Autodesk Fusion 360 part; units mm, degrees
(part 3 of 5)
  line L1736 (93.1413, -105.9405) -> (93.1413, -102.4186)
  line L1737 (93.1413, -102.4186) -> (79.4991, -102.4186)
  line L1738 (112.2258, -102.3705) -> (112.2394, -102.3841)
  line L1739 (112.2394, -102.3841) -> (112.2413, -102.3936)
  line L1740 (112.2413, -102.3936) -> (112.2413, -105.9655)
  line L1741 (112.2413, -105.9655) -> (112.2394, -105.9751)
  line L1742 (112.2394, -105.9751) -> (112.2258, -105.9886)
  line L1743 (112.2258, -105.9886) -> (112.2163, -105.9905)
  line L1744 (112.2163, -105.9905) -> (109.86, -105.9905)
  line L1745 (109.86, -105.9905) -> (109.86, -106.8585)
  line L1746 (109.86, -106.8585) -> (109.8581, -106.868)
  line L1747 (109.8581, -106.868) -> (109.8446, -106.8816)
  line L1748 (109.8446, -106.8816) -> (109.835, -106.8835)
  line L1749 (109.835, -106.8835) -> (107.1811, -106.8835)
  line L1750 (107.1811, -106.8835) -> (107.1811, -110.728)
  line L1751 (107.1811, -110.728) -> (107.1811, -111.9186)
  line L1752 (107.1811, -111.9186) -> (107.1792, -111.9282)
  line L1753 (107.1792, -111.9282) -> (107.1657, -111.9417)
  line L1754 (107.1657, -111.9417) -> (107.1561, -111.9436)
  line L1755 (107.1561, -111.9436) -> (102.6913, -111.9436)
  line L1756 (102.6913, -111.9436) -> (102.3936, -111.9436)
  line L1757 (102.3936, -111.9436) -> (102.384, -111.9417)
  line L1758 (102.384, -111.9417) -> (102.3705, -111.9282)
  line L1759 (102.3705, -111.9282) -> (102.3686, -111.9186)
  line L1760 (102.3686, -111.9186) -> (102.3686, -108.9671)
  line L1761 (102.3686, -108.9671) -> (100.9303, -108.9671)
  line L1762 (100.9303, -108.9671) -> (100.9303, -110.728)
  line L1763 (100.9303, -110.728) -> (100.9284, -110.7376)
  line L1764 (100.9284, -110.7376) -> (100.9149, -110.7511)
  line L1765 (100.9149, -110.7511) -> (100.9053, -110.753)
  line L1766 (100.9053, -110.753) -> (98.5241, -110.753)
  line L1767 (98.5241, -110.753) -> (98.5145, -110.7511)
  line L1768 (98.5145, -110.7511) -> (98.501, -110.7376)
  line L1769 (98.501, -110.7376) -> (98.4991, -110.728)
  line L1770 (98.4991, -110.728) -> (98.4991, -108.6694)
  line L1771 (98.4991, -108.6694) -> (96.1428, -108.6694)
  line L1772 (96.1428, -108.6694) -> (96.1333, -108.6675)
  line L1773 (96.1333, -108.6675) -> (96.1197, -108.654)
  line L1774 (96.1197, -108.654) -> (96.1178, -108.6444)
  line L1775 (96.1178, -108.6444) -> (96.1178, -105.3702)
  line L1776 (96.1178, -105.3702) -> (96.1197, -105.3606)
  line L1777 (96.1197, -105.3606) -> (96.1333, -105.3471)
  line L1778 (96.1333, -105.3471) -> (96.1428, -105.3452)
  line L1779 (96.1428, -105.3452) -> (98.4991, -105.3452)
  line L1780 (98.4991, -105.3452) -> (98.4991, -102.3936)
  line L1781 (98.4991, -102.3936) -> (98.501, -102.3841)
  line L1782 (98.501, -102.3841) -> (98.5145, -102.3705)
  line L1783 (98.5145, -102.3705) -> (98.5241, -102.3686)
  line L1784 (98.5241, -102.3686) -> (112.2163, -102.3686)
  line L1785 (112.2163, -102.3686) -> (112.2258, -102.3705)
  line L1786 (98.5491, -102.4186) -> (98.5491, -105.3702)
  line L1787 (98.5491, -105.3702) -> (98.5472, -105.3798)
  line L1788 (98.5472, -105.3798) -> (98.5336, -105.3933)
  line L1789 (98.5336, -105.3933) -> (98.5241, -105.3952)
  line L1790 (98.5241, -105.3952) -> (96.1678, -105.3952)
  line L1791 (96.1678, -105.3952) -> (96.1678, -108.6194)
  line L1792 (96.1678, -108.6194) -> (98.5241, -108.6194)
  line L1793 (98.5241, -108.6194) -> (98.5336, -108.6213)
  line L1794 (98.5336, -108.6213) -> (98.5472, -108.6348)
  line L1795 (98.5472, -108.6348) -> (98.5491, -108.6444)
  line L1796 (98.5491, -108.6444) -> (98.5491, -110.703)
  line L1797 (98.5491, -110.703) -> (100.8803, -110.703)
  line L1798 (100.8803, -110.703) -> (100.8803, -108.9421)
  line L1799 (100.8803, -108.9421) -> (100.8822, -108.9325)
  line L1800 (100.8822, -108.9325) -> (100.8958, -108.919)
  line L1801 (100.8958, -108.919) -> (100.9053, -108.9171)
  line L1802 (100.9053, -108.9171) -> (102.3936, -108.9171)
  line L1803 (102.3936, -108.9171) -> (102.4032, -108.919)
  line L1804 (102.4032, -108.919) -> (102.4167, -108.9325)
  line L1805 (102.4167, -108.9325) -> (102.4186, -108.9421)
  line L1806 (102.4186, -108.9421) -> (102.4186, -111.8936)
  line L1807 (102.4186, -111.8936) -> (102.6913, -111.8936)
  line L1808 (102.6913, -111.8936) -> (107.1311, -111.8936)
  line L1809 (107.1311, -111.8936) -> (107.1311, -110.728)
  line L1810 (107.1311, -110.728) -> (107.1311, -106.8585)
  line L1811 (107.1311, -106.8585) -> (107.133, -106.8489)
  line L1812 (107.133, -106.8489) -> (107.1465, -106.8354)
  line L1813 (107.1465, -106.8354) -> (107.1561, -106.8335)
  line L1814 (107.1561, -106.8335) -> (109.81, -106.8335)
  line L1815 (109.81, -106.8335) -> (109.81, -105.9655)
  line L1816 (109.81, -105.9655) -> (109.8119, -105.9559)
  line L1817 (109.8119, -105.9559) -> (109.8254, -105.9424)
  line L1818 (109.8254, -105.9424) -> (109.835, -105.9405)
  line L1819 (109.835, -105.9405) -> (112.1913, -105.9405)
  line L1820 (112.1913, -105.9405) -> (112.1913, -102.4186)
  line L1821 (112.1913, -102.4186) -> (98.5491, -102.4186)
  line L1822 (131.2758, -102.3705) -> (131.2894, -102.3841)
  line L1823 (131.2894, -102.3841) -> (131.2913, -102.3936)
  line L1824 (131.2913, -102.3936) -> (131.2913, -105.9655)
  line L1825 (131.2913, -105.9655) -> (131.2894, -105.9751)
  line L1826 (131.2894, -105.9751) -> (131.2758, -105.9886)
  line L1827 (131.2758, -105.9886) -> (131.2663, -105.9905)
  line L1828 (131.2663, -105.9905) -> (128.91, -105.9905)
  line L1829 (128.91, -105.9905) -> (128.91, -106.8585)
  line L1830 (128.91, -106.8585) -> (128.9081, -106.868)
  line L1831 (128.9081, -106.868) -> (128.8946, -106.8816)
  line L1832 (128.8946, -106.8816) -> (128.885, -106.8835)
  line L1833 (128.885, -106.8835) -> (126.2311, -106.8835)
  line L1834 (126.2311, -106.8835) -> (126.2311, -110.728)
  line L1835 (126.2311, -110.728) -> (126.2311, -111.9186)
  line L1836 (126.2311, -111.9186) -> (126.2292, -111.9282)
  line L1837 (126.2292, -111.9282) -> (126.2157, -111.9417)
  line L1838 (126.2157, -111.9417) -> (126.2061, -111.9436)
  line L1839 (126.2061, -111.9436) -> (121.7413, -111.9436)
  line L1840 (121.7413, -111.9436) -> (121.4436, -111.9436)
  line L1841 (121.4436, -111.9436) -> (121.434, -111.9417)
  line L1842 (121.434, -111.9417) -> (121.4205, -111.9282)
  line L1843 (121.4205, -111.9282) -> (121.4186, -111.9186)
  line L1844 (121.4186, -111.9186) -> (121.4186, -108.9671)
  line L1845 (121.4186, -108.9671) -> (119.9803, -108.9671)
  line L1846 (119.9803, -108.9671) -> (119.9803, -110.728)
  line L1847 (119.9803, -110.728) -> (119.9784, -110.7376)
  line L1848 (119.9784, -110.7376) -> (119.9649, -110.7511)
  line L1849 (119.9649, -110.7511) -> (119.9553, -110.753)
  line L1850 (119.9553, -110.753) -> (117.5741, -110.753)
  line L1851 (117.5741, -110.753) -> (117.5645, -110.7511)
  line L1852 (117.5645, -110.7511) -> (117.551, -110.7376)
  line L1853 (117.551, -110.7376) -> (117.5491, -110.728)
  line L1854 (117.5491, -110.728) -> (117.5491, -108.6694)
  line L1855 (117.5491, -108.6694) -> (115.1928, -108.6694)
  line L1856 (115.1928, -108.6694) -> (115.1833, -108.6675)
  line L1857 (115.1833, -108.6675) -> (115.1697, -108.654)
  line L1858 (115.1697, -108.654) -> (115.1678, -108.6444)
  line L1859 (115.1678, -108.6444) -> (115.1678, -105.3702)
  line L1860 (115.1678, -105.3702) -> (115.1697, -105.3606)
  line L1861 (115.1697, -105.3606) -> (115.1833, -105.3471)
  line L1862 (115.1833, -105.3471) -> (115.1928, -105.3452)
  line L1863 (115.1928, -105.3452) -> (117.5491, -105.3452)
  line L1864 (117.5491, -105.3452) -> (117.5491, -102.3936)
  line L1865 (117.5491, -102.3936) -> (117.551, -102.3841)
  line L1866 (117.551, -102.3841) -> (117.5645, -102.3705)
  line L1867 (117.5645, -102.3705) -> (117.5741, -102.3686)
  line L1868 (117.5741, -102.3686) -> (131.2663, -102.3686)
  line L1869 (131.2663, -102.3686) -> (131.2758, -102.3705)
  line L1870 (117.5991, -102.4186) -> (117.5991, -105.3702)
  line L1871 (117.5991, -105.3702) -> (117.5972, -105.3798)
  line L1872 (117.5972, -105.3798) -> (117.5836, -105.3933)
  line L1873 (117.5836, -105.3933) -> (117.5741, -105.3952)
  line L1874 (117.5741, -105.3952) -> (115.2178, -105.3952)
  line L1875 (115.2178, -105.3952) -> (115.2178, -108.6194)
  line L1876 (115.2178, -108.6194) -> (117.5741, -108.6194)
  line L1877 (117.5741, -108.6194) -> (117.5836, -108.6213)
  line L1878 (117.5836, -108.6213) -> (117.5972, -108.6348)
  line L1879 (117.5972, -108.6348) -> (117.5991, -108.6444)
  line L1880 (117.5991, -108.6444) -> (117.5991, -110.703)
  line L1881 (117.5991, -110.703) -> (119.9303, -110.703)
  line L1882 (119.9303, -110.703) -> (119.9303, -108.9421)
  line L1883 (119.9303, -108.9421) -> (119.9322, -108.9325)
  line L1884 (119.9322, -108.9325) -> (119.9458, -108.919)
  line L1885 (119.9458, -108.919) -> (119.9553, -108.9171)
  line L1886 (119.9553, -108.9171) -> (121.4436, -108.9171)
  line L1887 (121.4436, -108.9171) -> (121.4532, -108.919)
  line L1888 (121.4532, -108.919) -> (121.4667, -108.9325)
  line L1889 (121.4667, -108.9325) -> (121.4686, -108.9421)
  line L1890 (121.4686, -108.9421) -> (121.4686, -111.8936)
  line L1891 (121.4686, -111.8936) -> (121.7413, -111.8936)
  line L1892 (121.7413, -111.8936) -> (126.1811, -111.8936)
  line L1893 (126.1811, -111.8936) -> (126.1811, -110.728)
  line L1894 (126.1811, -110.728) -> (126.1811, -106.8585)
  line L1895 (126.1811, -106.8585) -> (126.183, -106.8489)
  line L1896 (126.183, -106.8489) -> (126.1965, -106.8354)
  line L1897 (126.1965, -106.8354) -> (126.2061, -106.8335)
  line L1898 (126.2061, -106.8335) -> (128.86, -106.8335)
  line L1899 (128.86, -106.8335) -> (128.86, -105.9655)
  line L1900 (128.86, -105.9655) -> (128.8619, -105.9559)
  line L1901 (128.8619, -105.9559) -> (128.8754, -105.9424)
  line L1902 (128.8754, -105.9424) -> (128.885, -105.9405)
  line L1903 (128.885, -105.9405) -> (131.2413, -105.9405)
  line L1904 (131.2413, -105.9405) -> (131.2413, -102.4186)
  line L1905 (131.2413, -102.4186) -> (117.5991, -102.4186)
  line L1906 (150.3258, -102.3705) -> (150.3394, -102.3841)
  line L1907 (150.3394, -102.3841) -> (150.3413, -102.3936)
  line L1908 (150.3413, -102.3936) -> (150.3413, -105.9655)
  line L1909 (150.3413, -105.9655) -> (150.3394, -105.9751)
  line L1910 (150.3394, -105.9751) -> (150.3258, -105.9886)
  line L1911 (150.3258, -105.9886) -> (150.3163, -105.9905)
  line L1912 (150.3163, -105.9905) -> (147.96, -105.9905)
  line L1913 (147.96, -105.9905) -> (147.96, -106.8585)
  line L1914 (147.96, -106.8585) -> (147.9581, -106.868)
  line L1915 (147.9581, -106.868) -> (147.9446, -106.8816)
  line L1916 (147.9446, -106.8816) -> (147.935, -106.8835)
  line L1917 (147.935, -106.8835) -> (145.2811, -106.8835)
  line L1918 (145.2811, -106.8835) -> (145.2811, -110.728)
  line L1919 (145.2811, -110.728) -> (145.2811, -111.9186)
  line L1920 (145.2811, -111.9186) -> (145.2792, -111.9282)
  line L1921 (145.2792, -111.9282) -> (145.2657, -111.9417)
  line L1922 (145.2657, -111.9417) -> (145.2561, -111.9436)
  line L1923 (145.2561, -111.9436) -> (140.7913, -111.9436)
  line L1924 (140.7913, -111.9436) -> (140.4936, -111.9436)
  line L1925 (140.4936, -111.9436) -> (140.484, -111.9417)
  line L1926 (140.484, -111.9417) -> (140.4705, -111.9282)
  line L1927 (140.4705, -111.9282) -> (140.4686, -111.9186)
  line L1928 (140.4686, -111.9186) -> (140.4686, -108.9671)
  line L1929 (140.4686, -108.9671) -> (139.0303, -108.9671)
  line L1930 (139.0303, -108.9671) -> (139.0303, -110.728)
  line L1931 (139.0303, -110.728) -> (139.0284, -110.7376)
  line L1932 (139.0284, -110.7376) -> (139.0149, -110.7511)
  line L1933 (139.0149, -110.7511) -> (139.0053, -110.753)
  line L1934 (139.0053, -110.753) -> (136.6241, -110.753)
  line L1935 (136.6241, -110.753) -> (136.6145, -110.7511)
  line L1936 (136.6145, -110.7511) -> (136.601, -110.7376)
  line L1937 (136.601, -110.7376) -> (136.5991, -110.728)
  line L1938 (136.5991, -110.728) -> (136.5991, -108.6694)
  line L1939 (136.5991, -108.6694) -> (134.2428, -108.6694)
  line L1940 (134.2428, -108.6694) -> (134.2333, -108.6675)
  line L1941 (134.2333, -108.6675) -> (134.2197, -108.654)
  line L1942 (134.2197, -108.654) -> (134.2178, -108.6444)
  line L1943 (134.2178, -108.6444) -> (134.2178, -105.3702)
  line L1944 (134.2178, -105.3702) -> (134.2197, -105.3606)
  line L1945 (134.2197, -105.3606) -> (134.2333, -105.3471)
  line L1946 (134.2333, -105.3471) -> (134.2428, -105.3452)
  line L1947 (134.2428, -105.3452) -> (136.5991, -105.3452)
  line L1948 (136.5991, -105.3452) -> (136.5991, -102.3936)
  line L1949 (136.5991, -102.3936) -> (136.601, -102.3841)
  line L1950 (136.601, -102.3841) -> (136.6145, -102.3705)
  line L1951 (136.6145, -102.3705) -> (136.6241, -102.3686)
  line L1952 (136.6241, -102.3686) -> (150.3163, -102.3686)
  line L1953 (150.3163, -102.3686) -> (150.3258, -102.3705)
  line L1954 (136.6491, -102.4186) -> (136.6491, -105.3702)
  line L1955 (136.6491, -105.3702) -> (136.6472, -105.3798)
  line L1956 (136.6472, -105.3798) -> (136.6336, -105.3933)
  line L1957 (136.6336, -105.3933) -> (136.6241, -105.3952)
  line L1958 (136.6241, -105.3952) -> (134.2678, -105.3952)
  line L1959 (134.2678, -105.3952) -> (134.2678, -108.6194)
  line L1960 (134.2678, -108.6194) -> (136.6241, -108.6194)
  line L1961 (136.6241, -108.6194) -> (136.6336, -108.6213)
  line L1962 (136.6336, -108.6213) -> (136.6472, -108.6348)
  line L1963 (136.6472, -108.6348) -> (136.6491, -108.6444)
  line L1964 (136.6491, -108.6444) -> (136.6491, -110.703)
  line L1965 (136.6491, -110.703) -> (138.9803, -110.703)
  line L1966 (138.9803, -110.703) -> (138.9803, -108.9421)
  line L1967 (138.9803, -108.9421) -> (138.9822, -108.9325)
  line L1968 (138.9822, -108.9325) -> (138.9958, -108.919)
  line L1969 (138.9958, -108.919) -> (139.0053, -108.9171)
  line L1970 (139.0053, -108.9171) -> (140.4936, -108.9171)
  line L1971 (140.4936, -108.9171) -> (140.5032, -108.919)
  line L1972 (140.5032, -108.919) -> (140.5167, -108.9325)
  line L1973 (140.5167, -108.9325) -> (140.5186, -108.9421)
  line L1974 (140.5186, -108.9421) -> (140.5186, -111.8936)
  line L1975 (140.5186, -111.8936) -> (140.7913, -111.8936)
  line L1976 (140.7913, -111.8936) -> (145.2311, -111.8936)
  line L1977 (145.2311, -111.8936) -> (145.2311, -110.728)
  line L1978 (145.2311, -110.728) -> (145.2311, -106.8585)
  line L1979 (145.2311, -106.8585) -> (145.233, -106.8489)
  line L1980 (145.233, -106.8489) -> (145.2465, -106.8354)
  line L1981 (145.2465, -106.8354) -> (145.2561, -106.8335)
  line L1982 (145.2561, -106.8335) -> (147.91, -106.8335)
  line L1983 (147.91, -106.8335) -> (147.91, -105.9655)
  line L1984 (147.91, -105.9655) -> (147.9119, -105.9559)
  line L1985 (147.9119, -105.9559) -> (147.9254, -105.9424)
  line L1986 (147.9254, -105.9424) -> (147.935, -105.9405)
  line L1987 (147.935, -105.9405) -> (150.2913, -105.9405)
  line L1988 (150.2913, -105.9405) -> (150.2913, -102.4186)
  line L1989 (150.2913, -102.4186) -> (136.6491, -102.4186)
  line L1990 (62.5173, -109.2167) -> (62.5309, -109.2302)
  line L1991 (62.5309, -109.2302) -> (62.5328, -109.2398)
  line L1992 (62.5328, -109.2398) -> (62.5328, -110.728)
  line L1993 (62.5328, -110.728) -> (62.5309, -110.7376)
  line L1994 (62.5309, -110.7376) -> (62.5173, -110.7511)
  line L1995 (62.5173, -110.7511) -> (62.5078, -110.753)
  line L1996 (62.5078, -110.753) -> (61.0195, -110.753)
  line L1997 (61.0195, -110.753) -> (61.0099, -110.7511)
  line L1998 (61.0099, -110.7511) -> (60.9964, -110.7376)
  line L1999 (60.9964, -110.7376) -> (60.9945, -110.728)
  line L2000 (60.9945, -110.728) -> (60.9945, -109.2398)
  line L2001 (60.9945, -109.2398) -> (60.9964, -109.2302)
  line L2002 (60.9964, -109.2302) -> (61.0099, -109.2167)
  line L2003 (61.0099, -109.2167) -> (61.0195, -109.2148)
  line L2004 (61.0195, -109.2148) -> (62.5078, -109.2148)
  line L2005 (62.5078, -109.2148) -> (62.5173, -109.2167)
  line L2006 (61.0445, -109.2648) -> (61.0445, -110.703)
  line L2007 (61.0445, -110.703) -> (62.4828, -110.703)
  line L2008 (62.4828, -110.703) -> (62.4828, -109.2648)
  line L2009 (62.4828, -109.2648) -> (61.0445, -109.2648)
  line L2010 (67.5775, -109.2167) -> (67.591, -109.2302)
  line L2011 (67.591, -109.2302) -> (67.5929, -109.2398)
  line L2012 (67.5929, -109.2398) -> (67.5929, -110.728)
  line L2013 (67.5929, -110.728) -> (67.591, -110.7376)
  line L2014 (67.591, -110.7376) -> (67.5775, -110.7511)
  line L2015 (67.5775, -110.7511) -> (67.5679, -110.753)
  line L2016 (67.5679, -110.753) -> (66.0796, -110.753)
  line L2017 (66.0796, -110.753) -> (66.0701, -110.7511)
  line L2018 (66.0701, -110.7511) -> (66.0565, -110.7376)
  line L2019 (66.0565, -110.7376) -> (66.0546, -110.728)
  line L2020 (66.0546, -110.728) -> (66.0546, -109.2398)
  line L2021 (66.0546, -109.2398) -> (66.0565, -109.2302)
  line L2022 (66.0565, -109.2302) -> (66.0701, -109.2167)
  line L2023 (66.0701, -109.2167) -> (66.0796, -109.2148)
  line L2024 (66.0796, -109.2148) -> (67.5679, -109.2148)
  line L2025 (67.5679, -109.2148) -> (67.5775, -109.2167)
  line L2026 (66.1046, -109.2648) -> (66.1046, -110.703)
  line L2027 (66.1046, -110.703) -> (67.5429, -110.703)
  line L2028 (67.5429, -110.703) -> (67.5429, -109.2648)
  line L2029 (67.5429, -109.2648) -> (66.1046, -109.2648)
  line L2030 (90.9961, -108.3402) -> (91.2008, -108.3951)
  line L2031 (91.2008, -108.3951) -> (91.3928, -108.4846)
  line L2032 (91.3928, -108.4846) -> (91.5664, -108.6062)
  line L2033 (91.5664, -108.6062) -> (91.7162, -108.756)
  line L2034 (91.7162, -108.756) -> (91.8378, -108.9296)
  line L2035 (91.8378, -108.9296) -> (91.9273, -109.1216)
  line L2036 (91.9273, -109.1216) -> (91.9822, -109.3263)
  line L2037 (91.9822, -109.3263) -> (92.0006, -109.5374)
  line L2038 (92.0006, -109.5374) -> (91.9822, -109.7485)
  line L2039 (91.9822, -109.7485) -> (91.9273, -109.9531)
  line L2040 (91.9273, -109.9531) -> (91.8378, -110.1452)
  line L2041 (91.8378, -110.1452) -> (91.7162, -110.3188)
  line L2042 (91.7162, -110.3188) -> (91.5664, -110.4686)
  line L2043 (91.5664, -110.4686) -> (91.3928, -110.5901)
  line L2044 (91.3928, -110.5901) -> (91.2008, -110.6797)
  line L2045 (91.2008, -110.6797) -> (90.9961, -110.7345)
  line L2046 (90.9961, -110.7345) -> (90.785, -110.753)
  line L2047 (90.785, -110.753) -> (90.5739, -110.7345)
  line L2048 (90.5739, -110.7345) -> (90.3692, -110.6797)
  line L2049 (90.3692, -110.6797) -> (90.1772, -110.5901)
  line L2050 (90.1772, -110.5901) -> (90.0036, -110.4686)
  line L2051 (90.0036, -110.4686) -> (89.8538, -110.3188)
  line L2052 (89.8538, -110.3188) -> (89.7322, -110.1452)
  line L2053 (89.7322, -110.1452) -> (89.6427, -109.9531)
  line L2054 (89.6427, -109.9531) -> (89.5879, -109.7485)
  line L2055 (89.5879, -109.7485) -> (89.5694, -109.5374)
  line L2056 (89.5694, -109.5374) -> (89.5879, -109.3263)
  line L2057 (89.5879, -109.3263) -> (89.6427, -109.1216)
  line L2058 (89.6427, -109.1216) -> (89.7322, -108.9296)
  line L2059 (89.7322, -108.9296) -> (89.8538, -108.756)
  line L2060 (89.8538, -108.756) -> (90.0036, -108.6062)
  line L2061 (90.0036, -108.6062) -> (90.1772, -108.4846)
  line L2062 (90.1772, -108.4846) -> (90.3692, -108.3951)
  line L2063 (90.3692, -108.3951) -> (90.5739, -108.3402)
  line L2064 (90.5739, -108.3402) -> (90.785, -108.3218)
  line L2065 (90.785, -108.3218) -> (90.9961, -108.3402)
  line L2066 (89.6343, -109.7525) -> (89.6934, -109.9603)
  line L2067 (89.6934, -109.9603) -> (89.7897, -110.1536)
  line L2068 (89.7897, -110.1536) -> (89.9199, -110.326)
  line L2069 (89.9199, -110.326) -> (90.0796, -110.4715)
  line L2070 (90.0796, -110.4715) -> (90.2632, -110.5853)
  line L2071 (90.2632, -110.5853) -> (90.4647, -110.6633)
  line L2072 (90.4647, -110.6633) -> (90.677, -110.703)
  line L2073 (90.677, -110.703) -> (90.893, -110.703)
  line L2074 (90.893, -110.703) -> (91.1054, -110.6633)
  line L2075 (91.1054, -110.6633) -> (91.3068, -110.5853)
  line L2076 (91.3068, -110.5853) -> (91.4905, -110.4715)
  line L2077 (91.4905, -110.4715) -> (91.6501, -110.326)
  line L2078 (91.6501, -110.326) -> (91.7803, -110.1536)
  line L2079 (91.7803, -110.1536) -> (91.8766, -109.9603)
  line L2080 (91.8766, -109.9603) -> (91.9357, -109.7525)
  line L2081 (91.9357, -109.7525) -> (91.9556, -109.5374)
  line L2082 (91.9556, -109.5374) -> (91.9357, -109.3223)
  line L2083 (91.9357, -109.3223) -> (91.8766, -109.1145)
  line L2084 (91.8766, -109.1145) -> (91.7803, -108.9211)
  line L2085 (91.7803, -108.9211) -> (91.6501, -108.7487)
  line L2086 (91.6501, -108.7487) -> (91.4905, -108.6032)
  line L2087 (91.4905, -108.6032) -> (91.3068, -108.4895)
  line L2088 (91.3068, -108.4895) -> (91.1054, -108.4114)
  line L2089 (91.1054, -108.4114) -> (90.893, -108.3718)
  line L2090 (90.893, -108.3718) -> (90.677, -108.3718)
  line L2091 (90.677, -108.3718) -> (90.4647, -108.4114)
  line L2092 (90.4647, -108.4114) -> (90.2632, -108.4895)
  line L2093 (90.2632, -108.4895) -> (90.0796, -108.6032)
  line L2094 (90.0796, -108.6032) -> (89.9199, -108.7487)
  line L2095 (89.9199, -108.7487) -> (89.7897, -108.9211)
  line L2096 (89.7897, -108.9211) -> (89.6934, -109.1145)
  line L2097 (89.6934, -109.1145) -> (89.6343, -109.3223)
  line L2098 (89.6343, -109.3223) -> (89.6144, -109.5374)
  line L2099 (89.6144, -109.5374) -> (89.6343, -109.7525)
  line L2100 (110.0461, -108.3402) -> (110.2508, -108.3951)
  line L2101 (110.2508, -108.3951) -> (110.4428, -108.4846)
  line L2102 (110.4428, -108.4846) -> (110.6164, -108.6062)
  line L2103 (110.6164, -108.6062) -> (110.7662, -108.756)
  line L2104 (110.7662, -108.756) -> (110.8878, -108.9296)
  line L2105 (110.8878, -108.9296) -> (110.9773, -109.1216)
  line L2106 (110.9773, -109.1216) -> (111.0322, -109.3263)
  line L2107 (111.0322, -109.3263) -> (111.0506, -109.5374)
  line L2108 (111.0506, -109.5374) -> (111.0322, -109.7485)
  line L2109 (111.0322, -109.7485) -> (110.9773, -109.9531)
  line L2110 (110.9773, -109.9531) -> (110.8878, -110.1452)
  line L2111 (110.8878, -110.1452) -> (110.7662, -110.3188)
  line L2112 (110.7662, -110.3188) -> (110.6164, -110.4686)
  line L2113 (110.6164, -110.4686) -> (110.4428, -110.5901)
  line L2114 (110.4428, -110.5901) -> (110.2508, -110.6797)
  line L2115 (110.2508, -110.6797) -> (110.0461, -110.7345)
  line L2116 (110.0461, -110.7345) -> (109.835, -110.753)
  line L2117 (109.835, -110.753) -> (109.6239, -110.7345)
  line L2118 (109.6239, -110.7345) -> (109.4192, -110.6797)
  line L2119 (109.4192, -110.6797) -> (109.2272, -110.5901)
  line L2120 (109.2272, -110.5901) -> (109.0536, -110.4686)
  line L2121 (109.0536, -110.4686) -> (108.9038, -110.3188)
  line L2122 (108.9038, -110.3188) -> (108.7822, -110.1452)
  line L2123 (108.7822, -110.1452) -> (108.6927, -109.9531)
  line L2124 (108.6927, -109.9531) -> (108.6379, -109.7485)
  line L2125 (108.6379, -109.7485) -> (108.6194, -109.5374)
  line L2126 (108.6194, -109.5374) -> (108.6379, -109.3263)
  line L2127 (108.6379, -109.3263) -> (108.6927, -109.1216)
  line L2128 (108.6927, -109.1216) -> (108.7822, -108.9296)
  line L2129 (108.7822, -108.9296) -> (108.9038, -108.756)
  line L2130 (108.9038, -108.756) -> (109.0536, -108.6062)
  line L2131 (109.0536, -108.6062) -> (109.2272, -108.4846)
  line L2132 (109.2272, -108.4846) -> (109.4192, -108.3951)
  line L2133 (109.4192, -108.3951) -> (109.6239, -108.3402)
  line L2134 (109.6239, -108.3402) -> (109.835, -108.3218)
  line L2135 (109.835, -108.3218) -> (110.0461, -108.3402)
  line L2136 (108.6843, -109.7525) -> (108.7434, -109.9603)
  line L2137 (108.7434, -109.9603) -> (108.8397, -110.1536)
  line L2138 (108.8397, -110.1536) -> (108.9699, -110.326)
  line L2139 (108.9699, -110.326) -> (109.1296, -110.4715)
  line L2140 (109.1296, -110.4715) -> (109.3132, -110.5853)
  line L2141 (109.3132, -110.5853) -> (109.5147, -110.6633)
  line L2142 (109.5147, -110.6633) -> (109.727, -110.703)
  line L2143 (109.727, -110.703) -> (109.943, -110.703)
  line L2144 (109.943, -110.703) -> (110.1554, -110.6633)
  line L2145 (110.1554, -110.6633) -> (110.3568, -110.5853)
  line L2146 (110.3568, -110.5853) -> (110.5405, -110.4715)
  line L2147 (110.5405, -110.4715) -> (110.7001, -110.326)
  line L2148 (110.7001, -110.326) -> (110.8303, -110.1536)
  line L2149 (110.8303, -110.1536) -> (110.9266, -109.9603)
  line L2150 (110.9266, -109.9603) -> (110.9857, -109.7525)
  line L2151 (110.9857, -109.7525) -> (111.0056, -109.5374)
  line L2152 (111.0056, -109.5374) -> (110.9857, -109.3223)
  line L2153 (110.9857, -109.3223) -> (110.9266, -109.1145)
  line L2154 (110.9266, -109.1145) -> (110.8303, -108.9211)
  line L2155 (110.8303, -108.9211) -> (110.7001, -108.7487)
  line L2156 (110.7001, -108.7487) -> (110.5405, -108.6032)
  line L2157 (110.5405, -108.6032) -> (110.3568, -108.4895)
  line L2158 (110.3568, -108.4895) -> (110.1554, -108.4114)
  line L2159 (110.1554, -108.4114) -> (109.943, -108.3718)
  line L2160 (109.943, -108.3718) -> (109.727, -108.3718)
  line L2161 (109.727, -108.3718) -> (109.5147, -108.4114)
  line L2162 (109.5147, -108.4114) -> (109.3132, -108.4895)
  line L2163 (109.3132, -108.4895) -> (109.1296, -108.6032)
  line L2164 (109.1296, -108.6032) -> (108.9699, -108.7487)
  line L2165 (108.9699, -108.7487) -> (108.8397, -108.9211)
  line L2166 (108.8397, -108.9211) -> (108.7434, -109.1145)
  line L2167 (108.7434, -109.1145) -> (108.6843, -109.3223)
  line L2168 (108.6843, -109.3223) -> (108.6644, -109.5374)
  line L2169 (108.6644, -109.5374) -> (108.6843, -109.7525)
  line L2170 (129.0961, -108.3402) -> (129.3008, -108.3951)
  line L2171 (129.3008, -108.3951) -> (129.4928, -108.4846)
  line L2172 (129.4928, -108.4846) -> (129.6664, -108.6062)
  line L2173 (129.6664, -108.6062) -> (129.8162, -108.756)
  line L2174 (129.8162, -108.756) -> (129.9378, -108.9296)
  line L2175 (129.9378, -108.9296) -> (130.0273, -109.1216)
  line L2176 (130.0273, -109.1216) -> (130.0822, -109.3263)
  line L2177 (130.0822, -109.3263) -> (130.1006, -109.5374)
  line L2178 (130.1006, -109.5374) -> (130.0822, -109.7485)
  line L2179 (130.0822, -109.7485) -> (130.0273, -109.9531)
  line L2180 (130.0273, -109.9531) -> (129.9378, -110.1452)
  line L2181 (129.9378, -110.1452) -> (129.8162, -110.3188)
  line L2182 (129.8162, -110.3188) -> (129.6664, -110.4686)
  line L2183 (129.6664, -110.4686) -> (129.4928, -110.5901)
  line L2184 (129.4928, -110.5901) -> (129.3008, -110.6797)
  line L2185 (129.3008, -110.6797) -> (129.0961, -110.7345)
  line L2186 (129.0961, -110.7345) -> (128.885, -110.753)
  line L2187 (128.885, -110.753) -> (128.6739, -110.7345)
  line L2188 (128.6739, -110.7345) -> (128.4692, -110.6797)
  line L2189 (128.4692, -110.6797) -> (128.2772, -110.5901)
  line L2190 (128.2772, -110.5901) -> (128.1036, -110.4686)
  line L2191 (128.1036, -110.4686) -> (127.9538, -110.3188)
  line L2192 (127.9538, -110.3188) -> (127.8322, -110.1452)
  line L2193 (127.8322, -110.1452) -> (127.7427, -109.9531)
  line L2194 (127.7427, -109.9531) -> (127.6879, -109.7485)
  line L2195 (127.6879, -109.7485) -> (127.6694, -109.5374)
  line L2196 (127.6694, -109.5374) -> (127.6879, -109.3263)
  line L2197 (127.6879, -109.3263) -> (127.7427, -109.1216)
  line L2198 (127.7427, -109.1216) -> (127.8322, -108.9296)
  line L2199 (127.8322, -108.9296) -> (127.9538, -108.756)
  line L2200 (127.9538, -108.756) -> (128.1036, -108.6062)
  line L2201 (128.1036, -108.6062) -> (128.2772, -108.4846)
  line L2202 (128.2772, -108.4846) -> (128.4692, -108.3951)
  line L2203 (128.4692, -108.3951) -> (128.6739, -108.3402)
  line L2204 (128.6739, -108.3402) -> (128.885, -108.3218)
  line L2205 (128.885, -108.3218) -> (129.0961, -108.3402)
  line L2206 (127.7343, -109.7525) -> (127.7934, -109.9603)
  line L2207 (127.7934, -109.9603) -> (127.8897, -110.1536)
  line L2208 (127.8897, -110.1536) -> (128.0199, -110.326)
  line L2209 (128.0199, -110.326) -> (128.1796, -110.4715)
  line L2210 (128.1796, -110.4715) -> (128.3632, -110.5853)
  line L2211 (128.3632, -110.5853) -> (128.5647, -110.6633)
  line L2212 (128.5647, -110.6633) -> (128.777, -110.703)
  line L2213 (128.777, -110.703) -> (128.993, -110.703)
  line L2214 (128.993, -110.703) -> (129.2054, -110.6633)
  line L2215 (129.2054, -110.6633) -> (129.4068, -110.5853)
  line L2216 (129.4068, -110.5853) -> (129.5905, -110.4715)
  line L2217 (129.5905, -110.4715) -> (129.7501, -110.326)
  line L2218 (129.7501, -110.326) -> (129.8803, -110.1536)
  line L2219 (129.8803, -110.1536) -> (129.9766, -109.9603)
  line L2220 (129.9766, -109.9603) -> (130.0357, -109.7525)
  line L2221 (130.0357, -109.7525) -> (130.0556, -109.5374)
  line L2222 (130.0556, -109.5374) -> (130.0357, -109.3223)
  line L2223 (130.0357, -109.3223) -> (129.9766, -109.1145)
  line L2224 (129.9766, -109.1145) -> (129.8803, -108.9211)
  line L2225 (129.8803, -108.9211) -> (129.7501, -108.7487)
  line L2226 (129.7501, -108.7487) -> (129.5905, -108.6032)
  line L2227 (129.5905, -108.6032) -> (129.4068, -108.4895)
  line L2228 (129.4068, -108.4895) -> (129.2054, -108.4114)
  line L2229 (129.2054, -108.4114) -> (128.993, -108.3718)
  line L2230 (128.993, -108.3718) -> (128.777, -108.3718)
  line L2231 (128.777, -108.3718) -> (128.5647, -108.4114)
  line L2232 (128.5647, -108.4114) -> (128.3632, -108.4895)
  line L2233 (128.3632, -108.4895) -> (128.1796, -108.6032)
  line L2234 (128.1796, -108.6032) -> (128.0199, -108.7487)
  line L2235 (128.0199, -108.7487) -> (127.8897, -108.9211)
  line L2236 (127.8897, -108.9211) -> (127.7934, -109.1145)
  line L2237 (127.7934, -109.1145) -> (127.7343, -109.3223)
  line L2238 (127.7343, -109.3223) -> (127.7144, -109.5374)
  line L2239 (127.7144, -109.5374) -> (127.7343, -109.7525)
  line L2240 (148.1461, -108.3402) -> (148.3508, -108.3951)
  line L2241 (148.3508, -108.3951) -> (148.5428, -108.4846)
  line L2242 (148.5428, -108.4846) -> (148.7164, -108.6062)
  line L2243 (148.7164, -108.6062) -> (148.8662, -108.756)
  line L2244 (148.8662, -108.756) -> (148.9878, -108.9296)
  line L2245 (148.9878, -108.9296) -> (149.0773, -109.1216)
  line L2246 (149.0773, -109.1216) -> (149.1322, -109.3263)
  line L2247 (149.1322, -109.3263) -> (149.1506, -109.5374)
  line L2248 (149.1506, -109.5374) -> (149.1322, -109.7485)
  line L2249 (149.1322, -109.7485) -> (149.0773, -109.9531)
  line L2250 (149.0773, -109.9531) -> (148.9878, -110.1452)
  line L2251 (148.9878, -110.1452) -> (148.8662, -110.3188)
  line L2252 (148.8662, -110.3188) -> (148.7164, -110.4686)
  line L2253 (148.7164, -110.4686) -> (148.5428, -110.5901)
  line L2254 (148.5428, -110.5901) -> (148.3508, -110.6797)
  line L2255 (148.3508, -110.6797) -> (148.1461, -110.7345)
  line L2256 (148.1461, -110.7345) -> (147.935, -110.753)
  line L2257 (147.935, -110.753) -> (147.7239, -110.7345)
  line L2258 (147.7239, -110.7345) -> (147.5192, -110.6797)
  line L2259 (147.5192, -110.6797) -> (147.3272, -110.5901)
  line L2260 (147.3272, -110.5901) -> (147.1536, -110.4686)
  line L2261 (147.1536, -110.4686) -> (147.0038, -110.3188)
  line L2262 (147.0038, -110.3188) -> (146.8822, -110.1452)
  line L2263 (146.8822, -110.1452) -> (146.7927, -109.9531)
  line L2264 (146.7927, -109.9531) -> (146.7379, -109.7485)
  line L2265 (146.7379, -109.7485) -> (146.7194, -109.5374)
  line L2266 (146.7194, -109.5374) -> (146.7379, -109.3263)
  line L2267 (146.7379, -109.3263) -> (146.7927, -109.1216)
  line L2268 (146.7927, -109.1216) -> (146.8822, -108.9296)
  line L2269 (146.8822, -108.9296) -> (147.0038, -108.756)
  line L2270 (147.0038, -108.756) -> (147.1536, -108.6062)
  line L2271 (147.1536, -108.6062) -> (147.3272, -108.4846)
  line L2272 (147.3272, -108.4846) -> (147.5192, -108.3951)
  line L2273 (147.5192, -108.3951) -> (147.7239, -108.3402)
  line L2274 (147.7239, -108.3402) -> (147.935, -108.3218)
  line L2275 (147.935, -108.3218) -> (148.1461, -108.3402)
  line L2276 (146.7843, -109.7525) -> (146.8434, -109.9603)
  line L2277 (146.8434, -109.9603) -> (146.9397, -110.1536)
  line L2278 (146.9397, -110.1536) -> (147.0699, -110.326)
  line L2279 (147.0699, -110.326) -> (147.2296, -110.4715)
  line L2280 (147.2296, -110.4715) -> (147.4132, -110.5853)
  line L2281 (147.4132, -110.5853) -> (147.6147, -110.6633)
  line L2282 (147.6147, -110.6633) -> (147.827, -110.703)
  line L2283 (147.827, -110.703) -> (148.043, -110.703)
  line L2284 (148.043, -110.703) -> (148.2554, -110.6633)
  line L2285 (148.2554, -110.6633) -> (148.4568, -110.5853)
  line L2286 (148.4568, -110.5853) -> (148.6405, -110.4715)
  line L2287 (148.6405, -110.4715) -> (148.8001, -110.326)
  line L2288 (148.8001, -110.326) -> (148.9303, -110.1536)
  line L2289 (148.9303, -110.1536) -> (149.0266, -109.9603)
  line L2290 (149.0266, -109.9603) -> (149.0857, -109.7525)
  line L2291 (149.0857, -109.7525) -> (149.1056, -109.5374)
  line L2292 (149.1056, -109.5374) -> (149.0857, -109.3223)
  line L2293 (149.0857, -109.3223) -> (149.0266, -109.1145)
  line L2294 (149.0266, -109.1145) -> (148.9303, -108.9211)
  line L2295 (148.9303, -108.9211) -> (148.8001, -108.7487)
  line L2296 (148.8001, -108.7487) -> (148.6405, -108.6032)
  line L2297 (148.6405, -108.6032) -> (148.4568, -108.4895)
  line L2298 (148.4568, -108.4895) -> (148.2554, -108.4114)
  line L2299 (148.2554, -108.4114) -> (148.043, -108.3718)
  line L2300 (148.043, -108.3718) -> (147.827, -108.3718)
  line L2301 (147.827, -108.3718) -> (147.6147, -108.4114)
  line L2302 (147.6147, -108.4114) -> (147.4132, -108.4895)
  line L2303 (147.4132, -108.4895) -> (147.2296, -108.6032)
  line L2304 (147.2296, -108.6032) -> (147.0699, -108.7487)
  line L2305 (147.0699, -108.7487) -> (146.9397, -108.9211)
  line L2306 (146.9397, -108.9211) -> (146.8434, -109.1145)
  line L2307 (146.8434, -109.1145) -> (146.7843, -109.3223)
  line L2308 (146.7843, -109.3223) -> (146.7644, -109.5374)
  line L2309 (146.7644, -109.5374) -> (146.7843, -109.7525)
  line L2310 (67.0033, -106.3832) -> (67.0168, -106.3967)
  line L2311 (67.0168, -106.3967) -> (67.0187, -106.4062)
  line L2312 (67.0187, -106.4062) -> (67.0187, -107.9062)
  line L2313 (67.0187, -107.9062) -> (67.0168, -107.9158)
  line L2314 (67.0168, -107.9158) -> (67.0033, -107.9293)
  line L2315 (67.0033, -107.9293) -> (66.9938, -107.9313)
  line L2316 (66.9938, -107.9313) -> (61.5938, -107.9313)
  line L2317 (61.5938, -107.9313) -> (61.5842, -107.9293)
  line L2318 (61.5842, -107.9293) -> (61.5707, -107.9158)
  line L2319 (61.5707, -107.9158) -> (61.5688, -107.9062)
  line L2320 (61.5688, -107.9062) -> (61.5688, -106.4062)
  line L2321 (61.5688, -106.4062) -> (61.5707, -106.3967)
  line L2322 (61.5707, -106.3967) -> (61.5842, -106.3832)
  line L2323 (61.5842, -106.3832) -> (61.5938, -106.3813)
  line L2324 (61.5938, -106.3813) -> (66.9938, -106.3813)
  line L2325 (66.9938, -106.3813) -> (67.0033, -106.3832)
  line L2326 (61.6188, -106.4313) -> (61.6188, -107.8812)
  line L2327 (61.6188, -107.8813) -> (66.9688, -107.8813)
  line L2328 (66.9688, -107.8813) -> (66.9688, -106.4313)
  line L2329 (66.9688, -106.4313) -> (61.6187, -106.4313)
  line L2330 (67.8751, -94.0362) -> (67.8887, -94.0497)
  line L2331 (67.8887, -94.0497) -> (67.8906, -94.0593)
  line L2332 (67.8906, -94.0593) -> (67.8906, -95.2249)
  line L2333 (67.8906, -95.2249) -> (71.735, -95.2249)
  line L2334 (71.735, -95.2249) -> (71.7446, -95.2268)
  line L2335 (71.7446, -95.2268) -> (71.7581, -95.2403)
  line L2336 (71.7581, -95.2403) -> (71.76, -95.2499)
  line L2337 (71.76, -95.2499) -> (71.76, -98.8218)
  line L2338 (71.76, -98.8218) -> (71.7581, -98.8313)
  line L2339 (71.7581, -98.8313) -> (71.7446, -98.8449)
  line L2340 (71.7446, -98.8449) -> (71.735, -98.8468)
  line L2341 (71.735, -98.8468) -> (69.3788, -98.8468)
  line L2342 (69.3788, -98.8468) -> (69.3788, -99.7147)
  line L2343 (69.3788, -99.7147) -> (69.3769, -99.7243)
  line L2344 (69.3769, -99.7243) -> (69.3633, -99.7378)
  line L2345 (69.3633, -99.7378) -> (69.3538, -99.7397)
  line L2346 (69.3538, -99.7397) -> (66.6999, -99.7397)
  line L2347 (66.6999, -99.7397) -> (66.6999, -103.5842)
  line L2348 (66.6999, -103.5842) -> (66.6999, -104.7749)
  line L2349 (66.6999, -104.7749) -> (66.698, -104.7844)
  line L2350 (66.698, -104.7844) -> (66.6844, -104.798)
  line L2351 (66.6844, -104.798) -> (66.6749, -104.7999)
  line L2352 (66.6749, -104.7999) -> (62.21, -104.7999)
  line L2353 (62.21, -104.7999) -> (61.9124, -104.7999)
  line L2354 (61.9124, -104.7999) -> (61.9028, -104.798)
  line L2355 (61.9028, -104.798) -> (61.8893, -104.7844)
  line L2356 (61.8893, -104.7844) -> (61.8874, -104.7749)
  line L2357 (61.8874, -104.7749) -> (61.8874, -101.8233)
  line L2358 (61.8874, -101.8233) -> (60.4491, -101.8233)
  line L2359 (60.4491, -101.8233) -> (60.4491, -103.5843)
  line L2360 (60.4491, -103.5842) -> (60.4472, -103.5938)
  line L2361 (60.4472, -103.5938) -> (60.4336, -103.6073)
  line L2362 (60.4336, -103.6073) -> (60.4241, -103.6093)
  line L2363 (60.4241, -103.6093) -> (58.0678, -103.6093)
  line L2364 (58.0678, -103.6093) -> (58.0678, -104.1796)
  line L2365 (58.0678, -104.1796) -> (58.0659, -104.1891)
  line L2366 (58.0659, -104.1891) -> (58.0524, -104.2027)
  line L2367 (58.0524, -104.2027) -> (58.0428, -104.2046)
  line L2368 (58.0428, -104.2046) -> (55.364, -104.2046)
  line L2369 (55.364, -104.2046) -> (55.3544, -104.2027)
  line L2370 (55.3544, -104.2027) -> (55.3409, -104.1891)
  line L2371 (55.3409, -104.1891) -> (55.339, -104.1796)
  line L2372 (55.339, -104.1796) -> (55.339, -98.2264)
  line L2373 (55.339, -98.2264) -> (55.3409, -98.2169)
  line L2374 (55.3409, -98.2169) -> (55.3544, -98.2033)
  line L2375 (55.3544, -98.2033) -> (55.364, -98.2014)
  line L2376 (55.364, -98.2014) -> (58.0178, -98.2014)
  line L2377 (58.0178, -98.2014) -> (58.0178, -95.2499)
  line L2378 (58.0178, -95.2499) -> (58.0197, -95.2403)
  line L2379 (58.0197, -95.2403) -> (58.0333, -95.2268)
  line L2380 (58.0333, -95.2268) -> (58.0428, -95.2249)
  line L2381 (58.0428, -95.2249) -> (60.6968, -95.2249)
  line L2382 (60.6968, -95.2249) -> (60.6968, -94.0593)
  line L2383 (60.6968, -94.0593) -> (60.6987, -94.0497)
  line L2384 (60.6987, -94.0497) -> (60.7123, -94.0362)
  line L2385 (60.7123, -94.0362) -> (60.7218, -94.0343)
  line L2386 (60.7218, -94.0343) -> (67.8656, -94.0343)
  line L2387 (67.8656, -94.0343) -> (67.8751, -94.0362)
  line L2388 (60.7468, -94.0843) -> (60.7468, -95.2499)
  line L2389 (60.7468, -95.2499) -> (60.7449, -95.2594)
  line L2390 (60.7449, -95.2594) -> (60.7314, -95.273)
  line L2391 (60.7314, -95.273) -> (60.7218, -95.2749)
  line L2392 (60.7218, -95.2749) -> (58.0678, -95.2749)
  line L2393 (58.0678, -95.2749) -> (58.0678, -98.2264)
  line L2394 (58.0678, -98.2264) -> (58.0659, -98.236)
  line L2395 (58.0659, -98.236) -> (58.0524, -98.2495)
  line L2396 (58.0524, -98.2495) -> (58.0428, -98.2514)
  line L2397 (58.0428, -98.2514) -> (55.389, -98.2514)
  line L2398 (55.389, -98.2514) -> (55.389, -104.1546)
  line L2399 (55.389, -104.1546) -> (58.0178, -104.1546)
  line L2400 (58.0178, -104.1546) -> (58.0178, -103.5842)
  line L2401 (58.0178, -103.5842) -> (58.0197, -103.5747)
  line L2402 (58.0197, -103.5747) -> (58.0333, -103.5612)
  line L2403 (58.0333, -103.5612) -> (58.0428, -103.5593)
  line L2404 (58.0428, -103.5593) -> (60.3991, -103.5593)
  line L2405 (60.3991, -103.5593) -> (60.3991, -101.7983)
  line L2406 (60.3991, -101.7983) -> (60.401, -101.7887)
  line L2407 (60.401, -101.7887) -> (60.4145, -101.7752)
  line L2408 (60.4145, -101.7752) -> (60.4241, -101.7733)
  line L2409 (60.4241, -101.7733) -> (61.9124, -101.7733)
  line L2410 (61.9124, -101.7733) -> (61.9219, -101.7752)
  line L2411 (61.9219, -101.7752) -> (61.9355, -101.7887)
  line L2412 (61.9355, -101.7887) -> (61.9374, -101.7983)
  line L2413 (61.9374, -101.7983) -> (61.9374, -104.7499)
  line L2414 (61.9374, -104.7499) -> (62.21, -104.7499)
  line L2415 (62.21, -104.7499) -> (66.6499, -104.7499)
  line L2416 (66.6499, -104.7499) -> (66.6499, -103.5843)
  line L2417 (66.6499, -103.5842) -> (66.6499, -99.7147)
  line L2418 (66.6499, -99.7147) -> (66.6518, -99.7052)
  line L2419 (66.6518, -99.7052) -> (66.6653, -99.6916)
  line L2420 (66.6653, -99.6916) -> (66.6749, -99.6897)
  line L2421 (66.6749, -99.6897) -> (69.3288, -99.6897)
  line L2422 (69.3288, -99.6897) -> (69.3288, -98.8218)
  line L2423 (69.3288, -98.8218) -> (69.3307, -98.8122)
  line L2424 (69.3307, -98.8122) -> (69.3442, -98.7987)
  line L2425 (69.3442, -98.7987) -> (69.3538, -98.7968)
  line L2426 (69.3538, -98.7968) -> (71.71, -98.7968)
  line L2427 (71.71, -98.7968) -> (71.71, -95.2749)
  line L2428 (71.71, -95.2749) -> (67.8656, -95.2749)
  line L2429 (67.8656, -95.2749) -> (67.856, -95.273)
  line L2430 (67.856, -95.273) -> (67.8425, -95.2595)
  line L2431 (67.8425, -95.2595) -> (67.8425, -95.2595)
  line L2432 (67.8425, -95.2595) -> (67.8406, -95.2499)
  line L2433 (67.8406, -95.2499) -> (67.8406, -94.0843)
  line L2434 (67.8406, -94.0843) -> (60.7468, -94.0843)
  line L2435 (73.2329, -100.8823) -> (73.2465, -100.8958)
  line L2436 (73.2465, -100.8958) -> (73.2484, -100.9053)
  line L2437 (73.2484, -100.9053) -> (73.2484, -103.8819)
  line L2438 (73.2484, -103.8819) -> (73.2465, -103.8915)
  line L2439 (73.2465, -103.8915) -> (73.2329, -103.905)
  line L2440 (73.2329, -103.905) -> (73.2234, -103.9069)
  line L2441 (73.2234, -103.9069) -> (69.3538, -103.9069)
  line L2442 (69.3538, -103.9069) -> (69.1171, -103.8883)
  line L2443 (69.1171, -103.8883) -> (68.8862, -103.8328)
  line L2444 (68.8862, -103.8328) -> (68.6668, -103.742)
  line L2445 (68.6668, -103.742) -> (68.4644, -103.6179)
  line L2446 (68.4644, -103.6179) -> (68.2838, -103.4637)
  line L2447 (68.2838, -103.4637) -> (68.1296, -103.2831)
  line L2448 (68.1296, -103.2831) -> (68.0055, -103.0806)
  line L2449 (68.0055, -103.0806) -> (67.9146, -102.8613)
  line L2450 (67.9146, -102.8613) -> (67.8592, -102.6304)
  line L2451 (67.8592, -102.6304) -> (67.8406, -102.3936)
  line L2452 (67.8406, -102.3936) -> (67.8592, -102.1569)
  line L2453 (67.8592, -102.1569) -> (67.9146, -101.926)
  line L2454 (67.9146, -101.926) -> (68.0055, -101.7066)
  line L2455 (68.0055, -101.7066) -> (68.1296, -101.5041)
  line L2456 (68.1296, -101.5041) -> (68.2838, -101.3236)
  line L2457 (68.2838, -101.3236) -> (68.4644, -101.1694)
  line L2458 (68.4644, -101.1694) -> (68.6668, -101.0453)
  line L2459 (68.6668, -101.0453) -> (68.8862, -100.9544)
  line L2460 (68.8862, -100.9544) -> (69.1171, -100.899)
  line L2461 (69.1171, -100.899) -> (69.3538, -100.8804)
  line L2462 (69.3538, -100.8804) -> (69.3538, -100.8803)
  line L2463 (69.3538, -100.8803) -> (73.2234, -100.8803)
  line L2464 (73.2234, -100.8803) -> (73.2329, -100.8823)
  line L2465 (69.3538, -100.9303) -> (69.3538, -100.9303)
  line L2466 (69.3538, -100.9303) -> (69.2387, -100.9304)
  line L2467 (69.2387, -100.9304) -> (69.0112, -100.9664)
  line L2468 (69.0112, -100.9664) -> (68.7921, -101.0376)
  line L2469 (68.7921, -101.0376) -> (68.5869, -101.1421)
  line L2470 (68.5869, -101.1421) -> (68.4006, -101.2775)
  line L2471 (68.4006, -101.2775) -> (68.2377, -101.4404)
  line L2472 (68.2377, -101.4404) -> (68.1023, -101.6267)
  line L2473 (68.1023, -101.6267) -> (67.9978, -101.8319)
  line L2474 (67.9978, -101.8319) -> (67.9266, -102.051)
  line L2475 (67.9266, -102.051) -> (67.8906, -102.2785)
  line L2476 (67.8906, -102.2785) -> (67.8906, -102.5088)
  line L2477 (67.8906, -102.5088) -> (67.9266, -102.7363)
  line L2478 (67.9266, -102.7363) -> (67.9978, -102.9553)
  line L2479 (67.9978, -102.9553) -> (68.1023, -103.1606)
  line L2480 (68.1023, -103.1606) -> (68.2377, -103.3469)
  line L2481 (68.2377, -103.3469) -> (68.4006, -103.5098)
  line L2482 (68.4006, -103.5098) -> (68.5869, -103.6451)
  line L2483 (68.5869, -103.6451) -> (68.7921, -103.7497)
  line L2484 (68.7921, -103.7497) -> (69.0112, -103.8209)
  line L2485 (69.0112, -103.8209) -> (69.2387, -103.8569)
  line L2486 (69.2387, -103.8569) -> (69.3538, -103.8569)
  line L2487 (69.3538, -103.8569) -> (73.1984, -103.8569)
  line L2488 (73.1984, -103.8569) -> (73.1984, -100.9303)
  line L2489 (73.1984, -100.9303) -> (69.3538, -100.9303)
  line L2490 (107.4846, -94.477) -> (107.4981, -94.4905)
  line L2491 (107.4981, -94.4905) -> (107.5, -94.5001)
  line L2492 (107.5, -94.5001) -> (107.5, -96.0001)
  line L2493 (107.5, -96.0001) -> (107.4981, -96.0096)
  line L2494 (107.4981, -96.0096) -> (107.4846, -96.0232)
  line L2495 (107.4846, -96.0232) -> (107.475, -96.0251)
  line L2496 (107.475, -96.0251) -> (102.075, -96.0251)
  line L2497 (102.075, -96.0251) -> (102.0654, -96.0232)
  line L2498 (102.0654, -96.0232) -> (102.0519, -96.0096)
  line L2499 (102.0519, -96.0096) -> (102.05, -96.0001)
  line L2500 (102.05, -96.0001) -> (102.05, -94.5001)
  line L2501 (102.05, -94.5001) -> (102.0519, -94.4905)
  line L2502 (102.0519, -94.4905) -> (102.0654, -94.477)
  line L2503 (102.0654, -94.477) -> (102.075, -94.4751)
  line L2504 (102.075, -94.4751) -> (107.475, -94.4751)
  line L2505 (107.475, -94.4751) -> (107.4846, -94.477)
  line L2506 (102.1, -94.5251) -> (102.1, -95.9751)
  line L2507 (102.1, -95.9751) -> (107.45, -95.9751)
  line L2508 (107.45, -95.9751) -> (107.45, -94.5251)
  line L2509 (107.45, -94.5251) -> (102.1, -94.5251)
  line L2510 (126.5346, -94.477) -> (126.5481, -94.4905)
  line L2511 (126.5481, -94.4905) -> (126.55, -94.5001)
  line L2512 (126.55, -94.5001) -> (126.55, -96.0001)
  line L2513 (126.55, -96.0001) -> (126.5481, -96.0096)
  line L2514 (126.5481, -96.0096) -> (126.5346, -96.0232)
  line L2515 (126.5346, -96.0232) -> (126.525, -96.0251)
  line L2516 (126.525, -96.0251) -> (121.125, -96.0251)
  line L2517 (121.125, -96.0251) -> (121.1154, -96.0232)
  line L2518 (121.1154, -96.0232) -> (121.1019, -96.0096)
  line L2519 (121.1019, -96.0096) -> (121.1, -96.0001)
  line L2520 (121.1, -96.0001) -> (121.1, -94.5001)
  line L2521 (121.1, -94.5001) -> (121.1019, -94.4905)
  line L2522 (121.1019, -94.4905) -> (121.1154, -94.477)
  line L2523 (121.1154, -94.477) -> (121.125, -94.4751)
  line L2524 (121.125, -94.4751) -> (126.525, -94.4751)
  line L2525 (126.525, -94.4751) -> (126.5346, -94.477)
  line L2526 (121.15, -94.5251) -> (121.15, -95.9751)
  line L2527 (121.15, -95.9751) -> (126.5, -95.9751)
  line L2528 (126.5, -95.9751) -> (126.5, -94.5251)
  line L2529 (126.5, -94.5251) -> (121.15, -94.5251)
  line L2530 (88.4346, -94.4769) -> (88.4481, -94.4904)
  line L2531 (88.4481, -94.4904) -> (88.45, -94.5)
  line L2532 (88.45, -94.5) -> (88.45, -96)
  line L2533 (88.45, -96) -> (88.4481, -96.0096)
  line L2534 (88.4481, -96.0096) -> (88.4346, -96.0231)
  line L2535 (88.4346, -96.0231) -> (88.425, -96.025)
  line L2536 (88.425, -96.025) -> (83.025, -96.025)
  line L2537 (83.025, -96.025) -> (83.0154, -96.0231)
  line L2538 (83.0154, -96.0231) -> (83.0019, -96.0096)
  line L2539 (83.0019, -96.0096) -> (83, -96)
  line L2540 (83, -96) -> (83, -94.5)
  line L2541 (83, -94.5) -> (83.0019, -94.4904)
  line L2542 (83.0019, -94.4904) -> (83.0154, -94.4769)
  line L2543 (83.0154, -94.4769) -> (83.025, -94.475)
  line L2544 (83.025, -94.475) -> (88.425, -94.475)
  line L2545 (88.425, -94.475) -> (88.4346, -94.4769)
  line L2546 (83.05, -94.525) -> (83.05, -95.975)
  line L2547 (83.05, -95.975) -> (88.4, -95.975)
  line L2548 (88.4, -95.975) -> (88.4, -94.525)
  line L2549 (88.4, -94.525) -> (83.05, -94.525)
  line L2550 (145.5846, -94.4769) -> (145.5981, -94.4904)
  line L2551 (145.5981, -94.4904) -> (145.6, -94.5)
  line L2552 (145.6, -94.5) -> (145.6, -96)
  line L2553 (145.6, -96) -> (145.5981, -96.0096)
  line L2554 (145.5981, -96.0096) -> (145.5846, -96.0231)
  line L2555 (145.5846, -96.0231) -> (145.575, -96.025)
  line L2556 (145.575, -96.025) -> (140.175, -96.025)
  line L2557 (140.175, -96.025) -> (140.1654, -96.0231)
  line L2558 (140.1654, -96.0231) -> (140.1519, -96.0096)
  line L2559 (140.1519, -96.0096) -> (140.15, -96)
  line L2560 (140.15, -96) -> (140.15, -94.5)
  line L2561 (140.15, -94.5) -> (140.1519, -94.4904)
  line L2562 (140.1519, -94.4904) -> (140.1654, -94.4769)
  line L2563 (140.1654, -94.4769) -> (140.175, -94.475)
  line L2564 (140.175, -94.475) -> (145.575, -94.475)
  line L2565 (145.575, -94.475) -> (145.5846, -94.4769)
  line L2566 (140.2, -94.525) -> (140.2, -95.975)
  line L2567 (140.2, -95.975) -> (145.55, -95.975)
  line L2568 (145.55, -95.975) -> (145.55, -94.525)
  line L2569 (145.55, -94.525) -> (140.2, -94.525)
  line L2570 (112.2258, -83.3206) -> (112.2394, -83.3341)
  line L2571 (112.2394, -83.3341) -> (112.2413, -83.3437)
  line L2572 (112.2413, -83.3437) -> (112.2413, -86.9156)
  line L2573 (112.2413, -86.9156) -> (112.2394, -86.9252)
  line L2574 (112.2394, -86.9252) -> (112.2258, -86.9387)
  line L2575 (112.2258, -86.9387) -> (112.2163, -86.9406)
  line L2576 (112.2163, -86.9406) -> (109.86, -86.9406)
  line L2577 (109.86, -86.9406) -> (109.86, -87.8086)
  line L2578 (109.86, -87.8086) -> (109.8581, -87.8181)
  line L2579 (109.8581, -87.8181) -> (109.8446, -87.8316)
  line L2580 (109.8446, -87.8316) -> (109.835, -87.8336)
  line L2581 (109.835, -87.8336) -> (107.1811, -87.8336)
  line L2582 (107.1811, -87.8336) -> (107.1811, -91.6781)
  line L2583 (107.1811, -91.6781) -> (107.1811, -92.8687)
  line L2584 (107.1811, -92.8687) -> (107.1792, -92.8783)
  line L2585 (107.1792, -92.8783) -> (107.1657, -92.8918)
  line L2586 (107.1657, -92.8918) -> (107.1561, -92.8937)
  line L2587 (107.1561, -92.8937) -> (102.6913, -92.8937)
  line L2588 (102.6913, -92.8937) -> (102.3936, -92.8937)
  line L2589 (102.3936, -92.8937) -> (102.384, -92.8918)
  line L2590 (102.384, -92.8918) -> (102.3705, -92.8783)
  line L2591 (102.3705, -92.8783) -> (102.3686, -92.8687)
  line L2592 (102.3686, -92.8687) -> (102.3686, -89.9171)
  line L2593 (102.3686, -89.9171) -> (100.9303, -89.9171)
  line L2594 (100.9303, -89.9171) -> (100.9303, -91.6781)
  line L2595 (100.9303, -91.6781) -> (100.9284, -91.6876)